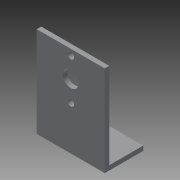
# Autodesk Inventor part: motor_support
Saved by Autodesk Inventor 2014 SP1 (Build 180222100, 222)
## iProperties
Created: 2014-09-21
Part Number: motor_support
Material: Générique
Document SubType Name: Modeling
Designer: astralien3000
Density: 1 g/cm^3
Appearance: Par défaut
d0: 40,000 mm
d1: 30,000 mm
d2: 15,000 mm
d3: 28,500 mm
d4: 7,000 mm
d7: 2,000 mm
d8: 0,00 deg
d9: 2,000 mm
d10: 15,000 mm
d11: 0,00 deg
d12: 3,000 mm
d13: 9,000 mm
Author: astralien3000
Autodesk Inventor part; units mm, degrees
ref_plane "YZ Plane" through (0, 0, 0) normal (1, 0, 0) x (0, 1, 0)
ref_plane "XZ Plane" through (0, 0, 0) normal (0, 1, 0) x (-1, 0, 0)
ref_plane "XY Plane" through (0, 0, 0) normal (0, 0, 1) x (1, 0, 0)
sketch "Esquisse1" plane through (0, 0, 0) normal (0, 1, 0) x (-1, 0, 0)
  line L0 (-15, 40) -> (15, 40)
  line L1 (15, 40) -> (15, 0)
  line L2 (15, 0) -> (-15, 0)
  line L3 (-15, 0) -> (-15, 40)
  line L4 (0, 0) -> (0, 40) construction
  circle A0 centre (0, 28.5) radius 3.5
  line L5 (0, 28.5) -> (-15, 28.5) construction
  line L6 (0, 28.5) -> (0, 32) construction
  line L7 (0, 28.5) -> (0, 40) construction
  circle A1 centre (0, 37.5) radius 1.5
  circle A2 centre (0, 19.5) radius 1.5
  dimension "d4" = 7
  dimension "d0" = 40
  dimension "d1" = 30
  dimension "d2" = 15
  dimension "d3" = 28.5
  dimension "d12" = 3
  dimension "d13" = 9
  constraints: 16 end point, 4 point on line, 2 centre point, 2 midpoint, 2 parallel, 2 perpendicular, 1 collinear, 1 horizontal, 1 vertical alignment, 3 other
  measures "d0" distance of L2.end L0.start
  measures "d1" distance of L0.start L0.end
  measures "d2" distance from line of L1 L4.start
  measures "d3" distance from line of L2 L5.start
  measures "d12" diameter of A1
  measures "d13" distance of A1.centre L5.start
extrude "Extrusion1" add sketch "Esquisse1" along normal blind 2
sketch "Esquisse2" plane through (0, 2, 0) normal (0, 1, 0) x (1, 0, 0)
  line L0 (15, -40) -> (15, 0) projected
  line L1 (-15, 0) -> (15, 0)
  line L2 (15, 0) -> (15, -2)
  line L3 (15, -2) -> (-15, -2)
  line L4 (-15, -2) -> (-15, 0)
  point P0 (0, 0)
  dimension "d9" = 2
  constraints: 8 end point, 2 parallel, 1 horizontal, 1 perpendicular, 1 point on line
  measures "d9" distance between parallel lines of L1 L3
extrude "Extrusion2" add sketch "Esquisse2" along normal blind 15
equation "\"d2\" = 0.5 * d1"
